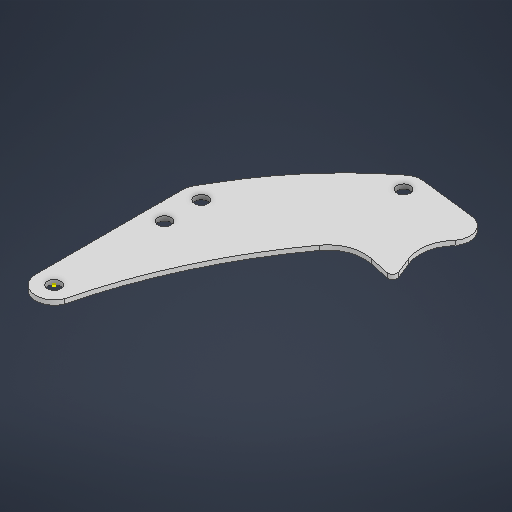
# Autodesk Inventor part: Lady Brown Tabs
Saved by Autodesk Inventor 2025 (Build 290162000, 162)
## iProperties
Created: 2024-12-29
Part Number: Lady Brown Tabs
Material: Generic
Document SubType Name: Modeling
Designer: Juan
Density: 1 g/cm^3
Appearance: Default
Author: Juan
Autodesk Inventor part; units mm, degrees
ref_plane "YZ Plane" through (0, 0, 0) normal (1, 0, 0) x (0, 1, 0)
ref_plane "XZ Plane" through (0, 0, 0) normal (0, 1, 0) x (-1, 0, 0)
ref_plane "XY Plane" through (0, 0, 0) normal (0, 0, 1) x (1, 0, 0)
sketch "Sketch1" plane through (0, 0, 0) normal (0, 1, 0) x (-1, 0, 0)
  circle A0 centre (0, 0) radius 2.3241
  line L0 (0, 0) -> (0, -38.1)
  circle A1 centre (0, -38.1) radius 2.3241
  line L1 (0, 0) -> (0, -38.1) construction
  line L2 (-6.35, 0) -> (-6.35, -38.1)
  line L3 (6.35, -38.1) -> (6.35, 0)
  arc A2 (6.35, 0) -> (-6.35, 0) centre (0, 0) ccw
  arc A3 (-6.35, -38.1) -> (6.35, -38.1) centre (0, -38.1) ccw
  line L4 (0, -38.1) -> (-15.9411, -38.1) construction
  line L5 (0, -31.75) -> (-15.9411, -31.75)
  line L6 (-15.9411, -44.45) -> (0, -44.45)
  arc A4 (0, -44.45) -> (0, -31.75) centre (0, -38.1) ccw
  arc A5 (-15.9411, -31.75) -> (-15.9411, -44.45) centre (-15.9411, -38.1) ccw
  line L7 (-5.9094, 2.3241) -> (-21.799, -35.6488)
  point P0 (0, -19.05)
  point P1 (-7.9706, -38.1)
  dimension "d0" = 4.6482
  dimension "d1" = 38.1
  dimension "d2" = 4.6482
  dimension "d3" = 12.7
  constraints: 20 end point, 10 point on circle, 9 tangent, 6 centre point, 3 equal length, 2 coincident, 2 midpoint, 1 perpendicular, 1 vertical
  measures "d0" diameter of A0
  measures "d1" distance of L0.start L0.end
  measures "d2" diameter of A1
  measures "d3" diameter of A3
extrude "Extrusion1" add sketch "Sketch1" along normal blind 1.5875
sketch "Sketch2" plane through (0, 1.5875, 0) normal (0, 1, 0) x (1, 0, 0)
  circle A0 centre (0, 38.1) radius 2.3241 projected
  line L0 (0, 38.1) -> (0, 31.75)
  line L1 (0, 31.75) -> (0, 92.71) construction
  line L2 (6.35, 38.1) -> (6.35, 86.36)
  line L3 (-6.35, 86.36) -> (-6.35, 38.1)
  arc A1 (-6.35, 38.1) -> (6.35, 38.1) centre (0, 38.1) ccw
  arc A2 (6.35, 86.36) -> (-6.35, 86.36) centre (0, 86.36) ccw
  line L4 (-6.35, 86.36) -> (57.15, 86.36) construction
  line L5 (0, 80.01) -> (50.8, 80.01)
  line L6 (50.8, 92.71) -> (0, 92.71)
  arc A3 (0, 92.71) -> (0, 80.01) centre (0, 86.36) ccw
  arc A4 (50.8, 80.01) -> (50.8, 92.71) centre (50.8, 86.36) ccw
  line L7 (-6.35, 38.1) -> (-6.35, 0) projected
  arc A5 (-6.35, 0) -> (5.9094, -2.3241) centre (0, 0) ccw projected
  line L8 (5.9094, -2.3241) -> (21.799, 35.6488) projected
  arc A6 (21.799, 35.6488) -> (15.9411, 44.45) centre (15.9411, 38.1) ccw projected
  line L9 (15.9411, 44.45) -> (0, 44.45) projected
  arc A7 (0, 44.45) -> (-6.35, 38.1) centre (0, 38.1) ccw projected
  circle A8 centre (0, 0) radius 2.3241 projected
  circle A9 centre (0, 38.1) radius 2.3241 projected
  line L10 (21.799, 35.6488) -> (55.9369, 82.6271)
  point P0 (0, 62.23)
  point P1 (25.4, 86.36)
  point P2 (0, 92.71)
  point P3 (6.35, 44.45)
  dimension "d6" = 6.35
  dimension "d7" = 60.96
  dimension "d10" = 63.5
  constraints: 20 end point, 13 point on circle, 9 tangent, 4 centre point, 4 point on line, 2 midpoint, 2 parallel, 2 vertical, 1 horizontal
  measures "d6" distance of L0.start L0.end
  measures "d7" distance of L0.end L1.end
  measures "d10" distance of L3.start L4.end
extrude "Extrusion2" add sketch "Sketch2" against normal blind 1.5875 contours A1 A7 L9 L2 | L9 A7 L3 A3 L5 L2 | L2 L5 A4 L10 A6 L9 | L5 A3 A2 L2 | L2 A2 L6 A4 L5
sketch "Sketch3" plane through (0, 1.5875, 0) normal (0, 1, 0) x (1, 0, 0)
  arc A0 (55.9369, 82.6271) -> (50.8, 92.71) centre (50.8, 86.36) ccw projected
  line L0 (5.9094, -2.3241) -> (21.799, 35.6488) projected
  arc A1 (55.9369, 82.6271) -> (5.9094, -2.3241) centre (174.4039, -44.3439) ccw
  line L1 (21.799, 35.6488) -> (55.9369, 82.6271) projected
  point P0 (0, 0)
  constraints: 2 point on circle, 1 centre point
extrude "Extrusion3" cut sketch "Sketch3" against normal blind 1.5875
sketch "Sketch4" plane through (0, 1.5875, 0) normal (0, 1, 0) x (1, 0, 0)
  line L0 (0, 92.71) -> (50.8, 92.71) projected
  line L1 (-6.35, 86.36) -> (-6.35, 0) projected
  arc A0 (30.6634, 92.71) -> (-6.35, 43.18) centre (81.4918, 16.1314) ccw
  arc A1 (55.9369, 82.6271) -> (5.9094, -2.3241) centre (174.4039, -44.3439) ccw projected
  arc A2 (55.9369, 82.6271) -> (50.8, 92.71) centre (50.8, 86.36) ccw projected
  line L2 (50.8, 92.71) -> (0, 92.71) projected
  arc A3 (0, 92.71) -> (-6.35, 86.36) centre (0, 86.36) ccw projected
  line L3 (-6.35, 86.36) -> (-6.35, 0) projected
  arc A4 (-6.35, 0) -> (5.9094, -2.3241) centre (0, 0) ccw projected
  circle A5 centre (0, 0) radius 2.3241 projected
  circle A6 centre (0, 38.1) radius 2.3241 projected
  constraints: 2 point on circle, 1 centre point, 1 midpoint, 1 point on line
extrude "Extrusion4" cut sketch "Sketch4" against normal blind 1.5875 contours L0 A0 L1 A3
sketch "Sketch5" plane through (0, 1.5875, 0) normal (0, 1, 0) x (1, 0, 0)
  point P0 (0, 0)
sketch "Sketch6" plane through (0, 1.5875, 0) normal (0, 1, 0) x (1, 0, 0)
  circle A0 centre (0, 38.1) radius 2.3241 projected
  line L0 (0, 38.1) -> (0, 50.8)
  circle A1 centre (0, 50.8) radius 2.3241
  point P0 (0, 0)
  dimension "d15" = 12.7
  dimension "d16" = 4.6482
  constraints: 2 end point, 1 centre point, 1 coincident, 1 vertical
  measures "d15" distance of L0.start L0.end
  measures "d16" diameter of A1
extrude "Extrusion5" cut sketch "Sketch6" against normal blind 1.5875 contours A1
sketch "Sketch7" plane through (0, 1.5875, 0) normal (0, 1, 0) x (1, 0, 0)
  circle A0 centre (0, 50.8) radius 2.3241 projected
  circle A1 centre (0, 38.1) radius 2.3241
  arc A2 (6.2992, 38.1) -> (-6.2992, 38.1) centre (0, 38.1) ccw
  circle A3 centre (0, 38.1) radius 2.3241 projected
  line L0 (0, 50.8) -> (0, 88.9)
  arc A4 (35.4436, 84.1127) -> (5.3749, 48.0302) centre (101.5031, -1.5067) ccw
  arc A5 (31.75, 88.9) -> (0, 50.8) centre (101.5031, -1.5067) ccw
  arc A6 (31.75, 88.9) -> (0, 50.8) centre (101.5031, -1.5067) ccw construction
  arc A7 (28.0564, 93.6873) -> (-5.3749, 53.5698) centre (101.5031, -1.5067) ccw
  line L1 (0, 88.9) -> (31.75, 88.9)
  arc A8 (35.4436, 84.1127) -> (28.0564, 93.6873) centre (31.75, 88.9) ccw
  line L2 (0, 50.8) -> (6.2992, 50.8)
  circle A9 centre (0, 50.8) radius 2.3241
  arc A10 (6.2992, 50.8) -> (-6.2992, 50.8) centre (0, 50.8) ccw
  line L3 (-6.2992, 50.8) -> (0, 50.8)
  arc A11 (-5.3749, 53.5698) -> (5.3749, 48.0302) centre (0, 50.8) ccw
  line L4 (-6.2992, 38.1) -> (-6.2992, 50.8)
  line L5 (0, 38.1) -> (0, 50.8) construction
  line L6 (6.2992, 50.8) -> (6.2992, 38.1)
  circle A12 centre (0, 38.1) radius 2.3241
  circle A13 centre (31.75, 88.9) radius 2.3241
  point P0 (0, 0)
  point P1 (0, 44.45)
  point P2 (-4.5326, 55.1744)
  point P3 (6.2992, 49.7843)
  point P4 (0, 57.0992)
  point P5 (2.3241, 50.8)
  point P6 (0, 53.1241)
  dimension "d19" = 4.6482
  dimension "d40" = 4.6482
  constraints: 17 point on circle, 16 end point, 12 centre point, 1 coincident
  measures "d19" diameter of A1
  measures "d40" diameter of A13
extrude "Extrusion6" add sketch "Sketch7" against normal blind 1.5875 contours L2 L6 A4 A11 L3 A0 | L3 A11 A7 A10 L0 A0 | A10 A5 A13 L1 A7 A8 A4 L6 | A10 L0 A7 L1 A13 A5 | A11 A4 L6 A2 L4 L3 | L3 A10 A7 A11 | A10 A7 L0 | A13 L1 A5 | A5 L1 A13
sketch "Sketch8" plane through (0, 1.5875, 0) normal (0, 1, 0) x (1, 0, 0)
  circle A0 centre (0, 50.8) radius 2.3241 projected
  circle A1 centre (0, 38.1) radius 2.3241 projected
  circle A2 centre (0, 0) radius 2.3241 projected
  arc A3 (36.4452, 92.71) -> (28.0564, 93.6873) centre (31.75, 88.9) ccw projected
  arc A4 (28.0564, 93.6873) -> (-4.5326, 55.1744) centre (101.5031, -1.5067) ccw projected
  arc A5 (-4.5326, 55.1744) -> (-6.2992, 50.8) centre (0, 50.8) ccw projected
  line L0 (-6.2992, 50.8) -> (-6.2992, 43.3444) projected
  arc A6 (-6.2992, 43.3444) -> (-6.35, 43.18) centre (81.4918, 16.1314) ccw projected
  line L1 (-6.35, 43.18) -> (-6.35, 0) projected
  arc A7 (-6.35, 0) -> (5.9094, -2.3241) centre (0, 0) ccw projected
  arc A8 (55.9369, 82.6271) -> (5.9094, -2.3241) centre (174.4039, -44.3439) ccw projected
  arc A9 (55.9369, 82.6271) -> (50.8, 92.71) centre (50.8, 86.36) ccw projected
  line L2 (50.8, 92.71) -> (36.4452, 92.71) projected
  arc A10 (55.9369, 82.6271) -> (50.8, 92.71) centre (50.8, 86.36) ccw projected
  line L3 (51.4711, 92.6744) -> (32.4545, 94.9054)
  constraints: 2 end point, 2 point on circle, 1 tangent
extrude "Extrusion7" add sketch "Sketch8" against normal blind 1.5875 contours A3 L3 A9 L2
sketch "Sketch11" plane through (0, 1.5875, 0) normal (0, 1, 0) x (1, 0, 0)
  arc A0 (55.9369, 82.6271) -> (5.9094, -2.3241) centre (174.4039, -44.3439) ccw projected
  line L0 (38.9499, 64.3219) -> (56.735, 60.5286)
  line L1 (56.735, 60.5286) -> (50.1783, 76.9989)
  circle A1 centre (0, 50.8) radius 2.3241 projected
  circle A2 centre (0, 38.1) radius 2.3241 projected
  circle A3 centre (0, 0) radius 2.3241 projected
  arc A4 (32.4545, 94.9054) -> (28.0564, 93.6873) centre (31.75, 88.9) ccw projected
  arc A5 (28.0564, 93.6873) -> (-4.5326, 55.1744) centre (101.5031, -1.5067) ccw projected
  arc A6 (-4.5326, 55.1744) -> (-6.2992, 50.8) centre (0, 50.8) ccw projected
  line L2 (-6.2992, 50.8) -> (-6.2992, 43.3444) projected
  arc A7 (-6.2992, 43.3444) -> (-6.35, 43.18) centre (81.4918, 16.1314) ccw projected
  line L3 (-6.35, 43.18) -> (-6.35, 0) projected
  arc A8 (-6.35, 0) -> (5.9094, -2.3241) centre (0, 0) ccw projected
  arc A9 (55.9369, 82.6271) -> (5.9094, -2.3241) centre (174.4039, -44.3439) ccw projected
  arc A10 (55.9369, 82.6271) -> (51.4711, 92.6744) centre (50.8, 86.36) ccw projected
  line L4 (51.4711, 92.6744) -> (32.4545, 94.9054) projected
  constraints: 4 end point, 2 point on circle
extrude "Extrusion10" add sketch "Sketch11" against normal blind 1.5875 contours L1 L0 A0
fillet "Fillet4" radius 12.7 2 edges at (50.1783, 0.7937, -76.9989) (38.9499, 0.7937, -64.3219)
fillet "Fillet5" radius 1.5875 1 edges at (56.735, 0.7937, -60.5286)
extrude "Extrusion11" cut sketch "Sketch7" against normal blind 1.5875 contours A13 L1 A5 | A5 L1 A13
fillet "Fillet6" radius 127 1 edges at (-4.5326, 0.7937, -55.1744)
body "Solid1"
